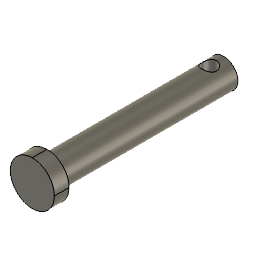
lock_pin (Autodesk Fusion 360 design; units mm, degrees)
part number: 2025-10-30-15-00-38-452
Autodesk Fusion 360 part; units mm, degrees
sketch "Sketch1" plane through (0, 0, 0) normal (0, 1, 0) x (1, 0, 0)
  circle A0 centre (0, -12.7) radius 2.4765
  dimension "d1" = 4.953
  measures "d1" diameter of A0
extrude "Extrude1" add sketch "Sketch1" along normal blind 30.48
hole "Hole1" at (0, 27.94, 15.1765) direction (0, 0, -1) diameter 2.54 depth 10.668 tip angle 118
sketch "Sketch2" plane through (0, 0, 0) normal (0, -1, 0) x (1, 0, 0)
  circle A0 centre (0, 12.7) radius 2.4765
  line L0 (-1.27, 11.43) -> (1.27, 11.43)
  line L1 (1.27, 11.43) -> (1.27, 13.97)
  line L2 (1.27, 13.97) -> (-1.27, 13.97)
  line L3 (-1.27, 13.97) -> (-1.27, 11.43)
  constraint horizontal L0
  constraint vertical L1
  constraint horizontal L2
  constraint vertical L3
extrude "Extrude2" add sketch "Sketch2" along normal blind 2.54 contours L0 L1 L2 L3
extrude "Extrude3" add 1 faces at (0.4233, -0.8467, 13.97) along direction (0, 0, 1) blind 2.54
extrude "Extrude4" add 1 faces at (-0.4233, -0.8467, 11.43) along direction (0, 0, -1) blind 2.54
extrude "Extrude5" add 1 faces at (-1.27, -1.6933, 11.9913) along direction (-1, 0, 0) blind 2.54
extrude "Extrude6" add 1 faces at (1.27, -1.6933, 11.9913) along direction (1, 0, 0) blind 2.54
fillet "Fillet1" radius 3.81 4 edges at (-3.81, -1.27, 16.51) (3.81, -1.27, 16.51) (3.81, -1.27, 8.89) (-3.81, -1.27, 8.89)
